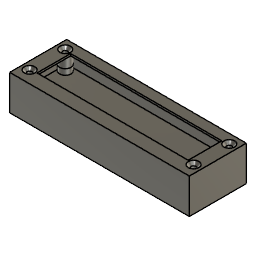
1601_display_case (Autodesk Fusion 360 design; units mm, degrees)
Autodesk Fusion 360 part; units mm, degrees
sketch "Sketch1" plane through (0, 0, 0) normal (0, 0, 1) x (1, 0, 0)
  line L0 (0, 0) -> (122, 0)
  line L1 (122, 0) -> (122, 33)
  line L2 (122, 33) -> (0, 33)
  line L3 (0, 33) -> (0, 0)
  line L4 (7.98, 33.5) -> (87.98, 33.5)
  line L5 (87.98, 33.5) -> (87.98, -2.5)
  line L6 (87.98, -2.5) -> (7.98, -2.5)
  line L7 (7.98, -2.5) -> (7.98, 33.5)
  circle A0 centre (3.5, 29) radius 1.75
  circle A1 centre (3.5, 4) radius 1.75
  circle A2 centre (118.5, 29) radius 1.75
  circle A3 centre (118.5, 4) radius 1.75
  line L8 (8, 28.27) -> (114, 28.27)
  line L9 (114, 28.27) -> (114, 4.73)
  line L10 (114, 4.73) -> (8, 4.73)
  line L11 (8, 4.73) -> (8, 28.27)
  line L12 (7.98, 33.5) -> (0, 33.5)
  line L13 (0, 33.5) -> (0, 33)
  line L14 (87.98, 33.5) -> (122, 33.5)
  line L15 (122, 33.5) -> (122, 33)
  line L16 (7.98, -2.5) -> (0, -2.5)
  line L17 (0, -2.5) -> (0, 0)
  line L18 (122, 0) -> (122, -2.5)
  line L19 (122, -2.5) -> (87.98, -2.5)
  circle A4 centre (3.5, 29) radius 4
  circle A5 centre (3.5, 4) radius 4
  circle A6 centre (118.5, 29) radius 4
  circle A7 centre (118.5, 4) radius 4
  line L20 (-2, 35.5) -> (124, 35.5)
  line L21 (124, 35.5) -> (124, -4.5)
  line L22 (124, -4.5) -> (-2, -4.5)
  line L23 (-2, -4.5) -> (-2, 35.5)
  line L24 (-2, 22) -> (7.98, 22)
  line L25 (7.98, 22) -> (7.98, 9)
  line L26 (7.98, 9) -> (-2, 9)
  line L27 (-2, 9) -> (-2, 22)
  point P0 (15.98, 31)
  dimension "d1" = 122
  dimension "d2" = 33
  dimension "d3" = 15.98
  dimension "d4" = 2
  dimension "d5" = 2.5
  dimension "d6" = 8
  dimension "d7" = 36
  dimension "d8" = 80
  dimension "d9" = 3.5
  dimension "d10" = 3.5
  dimension "d11" = 3.5
  dimension "d12" = 3.5
  dimension "d13" = 4
  dimension "d14" = 3.5
  dimension "d15" = 4
  dimension "d16" = 3.5
  dimension "d17" = 4
  dimension "d18" = 3.5
  dimension "d19" = 4
  dimension "d20" = 3.5
  dimension "d21" = 4.73
  dimension "d22" = 4.73
  dimension "d23" = 8
  dimension "d24" = 8
  dimension "d25" = 8
  dimension "d26" = 8
  dimension "d27" = 8
  dimension "d28" = 8
  dimension "d29" = 2
  dimension "d30" = 2
  dimension "d31" = 2
  dimension "d32" = 2
  dimension "d51" = 11.5
  dimension "d52" = 11.5
  constraint horizontal L0
  constraint vertical L1
  constraint horizontal L2
  constraint vertical L3
  constraint coincident L0.start L3.end
  constraint horizontal L4
  constraint vertical L5
  constraint horizontal L6
  constraint vertical L7
  constraint horizontal L8
  constraint vertical L9
  constraint horizontal L10
  constraint vertical L11
  constraint perpendicular L7 L12
  constraint perpendicular L2 L13
  constraint perpendicular L1 L14
  constraint perpendicular L2 L15
  constraint perpendicular L7 L16
  constraint perpendicular L0 L17
  constraint perpendicular L0 L18
  constraint perpendicular L5 L19
  constraint concentric A0 A4
  constraint concentric A1 A5
  constraint concentric A2 A6
  constraint concentric A3 A7
  constraint horizontal L20
  constraint vertical L21
  constraint horizontal L22
  constraint vertical L23
  constraint horizontal L24
  constraint vertical L25
  constraint horizontal L26
  constraint vertical L27
  constraint coincident L7 L25.end
  constraint coincident L23 L24.start
  measures "d1" distance of L0.start L0.end
  measures "d2" distance of L0.start L2.end
  measures "d3" distance of L3 P0
  measures "d4" distance of L2 P0
  measures "d5" distance of P0 L4
  measures "d6" distance of P0 L7
  measures "d7" distance of L4 L6
  measures "d8" distance of L5 L7
  measures "d9" diameter of A0
  measures "d10" diameter of A1
  measures "d11" diameter of A2
  measures "d12" diameter of A3
  measures "d13" distance of L2 A2.centre
  measures "d14" distance of L1 A2.centre
  measures "d15" distance of L0 A3.centre
  measures "d16" distance of L1 A3.centre
  measures "d17" distance of L2 A0.centre
  measures "d18" distance of L3 A0.centre
  measures "d19" distance of L0 A1.centre
  measures "d20" distance of L3 A1.centre
  measures "d21" distance of L2 L8
  measures "d22" distance of L0 L10
  measures "d23" distance of L1 L9
  measures "d24" distance of L3 L11
  measures "d25" diameter of A4
  measures "d26" diameter of A5
  measures "d27" diameter of A6
  measures "d28" diameter of A7
  measures "d29" distance of L1 L21
  measures "d30" distance of L6 L22
  measures "d31" distance of L4 L20
  measures "d32" distance of L3 L23
  measures "d51" distance of L16 L26
  measures "d52" distance of L12 L24
extrude "Extrude1" add sketch "Sketch1" along normal blind 9 contours L0 L3 A5 | L1 L3 L4 L6 L12 L13 L14 L15 L16 L17 L18 L19 A4 A5 A6 A7 L20 L21 L22 L23 L24 L26 | L0 L7 L16 L17 | L0 L3 L7 A5 L26 | L3 A5 | L3 A5 | L0 L2 L5 L7 L8 L10 L11 L25 | L0 L5 L6 L7 | L0 L1 L2 L5 L8 L9 L10 A6 A7 | L0 L5 L18 L19 | L3 L7 L24 L25 L26 | L3 L23 L24 L26 L27 | L0 L1 A7 | L1 A7 | L2 L3 L7 A4 L24 | L1 A7 | L2 L4 L5 L7 | L2 L7 L12 L13 | L3 A4 | L3 A4 | L1 A6 | L1 A6 | L2 L5 L14 L15 | L2 L3 A4 | L1 L2 A6 makes body 1
extrude "Extrude2" cut sketch "Sketch1" along normal blind 7.6 contours L0 L3 A5 | L0 L7 L16 L17 | L0 L3 L7 A5 L26 | L0 L2 L5 L7 L8 L10 L11 L25 | L0 L5 L6 L7 | L0 L1 L2 L5 L8 L9 L10 A6 A7 | L0 L5 L18 L19 | L3 L7 L24 L25 L26 | L0 L1 A7 | L2 L3 L7 A4 L24 | L2 L4 L5 L7 | L2 L7 L12 L13 | L2 L5 L14 L15 | L2 L3 A4 | L1 L2 A6 bodies 1
chamfer "Chamfer1" distance 2 angle 45 4 edges at (1.8684, 29.6328, 9) (116.8684, 29.6328, 9) (1.8684, 4.6328, 9) (116.8684, 4.6328, 9) on bodies 1
extrude "Extrude3" add sketch "Sketch1" against normal blind 15.6 contours L1 L3 L4 L6 L12 L13 L14 L15 L16 L17 L18 L19 A4 A5 A6 A7 L20 L21 L22 L23 L24 L26 | L3 A5 | L3 L23 L24 L26 L27 | L1 A7 | L3 A4 | L1 A6 picked at (-0.0807, 4.4709) picked at (122.072, 3.5067) picked at (-0.0807, 29.4709) picked at (122.072, 28.5067) bodies 1
sketch "Sketch2" plane through (-2, 0, 0) normal (-1, 0, 0) x (0, -1, 0)
  line L0 (4.5, -15.6) -> (4.5, 9)
  line L1 (4.5, 9) -> (-35.5, 9)
  line L2 (-35.5, 9) -> (-35.5, -15.6)
  line L3 (-35.5, -15.6) -> (4.5, -15.6)
  line L4 (-22, -4.9) -> (-9, -4.9)
  line L5 (-9, -4.9) -> (-9, -12.9)
  line L6 (-9, -12.9) -> (-22, -12.9)
  line L7 (-22, -12.9) -> (-22, -4.9)
  line L8 (4.5, 0) -> (-35.5, 0)
  dimension "d45" = 13.5
  dimension "d46" = 13.5
  dimension "d47" = 8
  dimension "d48" = 4.9
  constraint horizontal L4
  constraint vertical L5
  constraint horizontal L6
  constraint vertical L7
  measures "d45" distance of L0 L5
  measures "d46" distance of L2 L7
  measures "d47" distance of L4 L6
  measures "d48" distance of L4 L8
extrude "Extrude6" cut sketch "Sketch2" against normal blind 2 contours L4 L5 L6 L7 bodies 1
extrude "Extrude4" add sketch "Sketch1" against normal blind 6 separate body contours L0 L3 A5 | L0 L7 L16 L17 | L0 L3 L7 A5 L26 | L3 A5 | L0 L2 L5 L7 L8 L10 L11 L25 | L0 L5 L6 L7 | L0 L1 L2 L5 L8 L9 L10 A6 A7 | L0 L5 L18 L19 | L3 L7 L24 L25 L26 | L0 L1 A7 | L1 A7 | L5 L8 L10 L11 | L5 L8 L9 L10 | L2 L3 L7 A4 L24 | L2 L4 L5 L7 | L2 L7 L12 L13 | L3 A4 | L1 A6 | L2 L5 L14 L15 | L2 L3 A4 | L1 L2 A6 picked at (0.5833, 4) picked at (121.4167, 4) picked at (0.5833, 29) picked at (121.4167, 29) makes body 2
extrude "Extrude5" cut sketch "Sketch1" against normal blind 4 contours L0 L3 A5 | L0 L7 L16 L17 | L0 L3 L7 A5 L26 | L0 L2 L5 L7 L8 L10 L11 L25 | L0 L5 L6 L7 | L0 L1 L2 L5 L8 L9 L10 A6 A7 | L0 L5 L18 L19 | L3 L7 L24 L25 L26 | L0 L1 A7 | L5 L8 L10 L11 | L5 L8 L9 L10 | L2 L3 L7 A4 L24 | L2 L4 L5 L7 | L2 L7 L12 L13 | L2 L5 L14 L15 | L2 L3 A4 | L1 L2 A6 bodies 2
chamfer "Chamfer2" distance 1.8 angle 45 4 edges at (116.8684, 3.3672, -6) (1.8684, 3.3672, -6) (1.8684, 28.3672, -6) (116.8684, 28.3672, -6) on bodies 2
